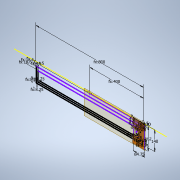
# Autodesk Inventor part: primary_coil_0R2_test_cut
Saved by Autodesk Inventor 2021 (Build 250183000, 183)
## iProperties
Created: 2021-01-20
Part Number: primary_coil_0R2_test_cut
Material: Generic
Document SubType Name: Modeling
Designer: phamv
Density: 1 g/cm^3
Appearance: Default
Author: phamv
Autodesk Inventor part; units mm, degrees
ref_plane "YZ Plane" through (0, 0, 0) normal (1, 0, 0) x (0, 1, 0)
sketch "Sketch1" plane through (0, 0, 0) normal (0, 0, 1) x (1, 0, 0)
  line L0 (-5, -4.3) -> (380, -4.3)
  line L1 (400, -24.3) -> (400, -120)
  line L2 (380, -140) -> (-400, -140)
  line L3 (-400, -140) -> (-400, -27.4)
  line L4 (-5, -4.3) -> (-5, -8.8)
  line L5 (-5, -8.8) -> (375.5, -8.8)
  line L6 (395.5, -28.8) -> (395.5, -115.5)
  line L7 (375.5, -135.5) -> (-395.5, -135.5)
  line L8 (-400, -27.4) -> (367.25, -27.4)
  line L9 (387.25, -47.4) -> (387.25, -107.25)
  line L10 (367.25, -127.25) -> (-387.25, -127.25)
  line L11 (-395.5, -135.5) -> (-395.5, -31.9)
  line L12 (-395.5, -31.9) -> (362.75, -31.9)
  line L13 (382.75, -51.9) -> (382.75, -102.75)
  line L14 (362.75, -122.75) -> (-382.75, -122.75)
  line L15 (-382.75, -122.75) -> (-382.75, -55)
  line L16 (-387.25, -127.25) -> (-387.25, -50.5)
  line L17 (-387.25, -50.5) -> (354.5, -50.5)
  line L18 (374.5, -70.5) -> (374.5, -94.5)
  line L19 (-382.75, -55) -> (350, -55)
  line L20 (370, -75) -> (370, -90)
  line L21 (350, -110) -> (-374.5, -110)
  line L22 (354.5, -114.5) -> (-374.5, -114.5)
  line L23 (-374.5, -114.5) -> (-374.5, -110)
  arc A0 (400, -24.3) -> (380, -4.3) centre (380, -24.3) ccw
  arc A1 (395.5, -28.8) -> (375.5, -8.8) centre (375.5, -28.8) ccw
  arc A2 (387.25, -47.4) -> (367.25, -27.4) centre (367.25, -47.4) ccw
  arc A3 (382.75, -51.9) -> (362.75, -31.9) centre (362.75, -51.9) ccw
  arc A4 (374.5, -70.5) -> (354.5, -50.5) centre (354.5, -70.5) ccw
  arc A5 (370, -75) -> (350, -55) centre (350, -75) ccw
  arc A6 (350, -110) -> (370, -90) centre (350, -90) ccw
  arc A7 (354.5, -114.5) -> (374.5, -94.5) centre (354.5, -94.5) ccw
  arc A8 (362.75, -122.75) -> (382.75, -102.75) centre (362.75, -102.75) ccw
  arc A9 (367.25, -127.25) -> (387.25, -107.25) centre (367.25, -107.25) ccw
  arc A10 (375.5, -135.5) -> (395.5, -115.5) centre (375.5, -115.5) ccw
  arc A11 (380, -140) -> (400, -120) centre (380, -120) ccw
  line L24 (323.0472, 0) -> (323.0472, -162)
  line L25 (323.0472, -162) -> (407.7972, -162)
  line L26 (407.7972, -162) -> (407.7972, 0)
  line L27 (407.7972, 0) -> (323.0472, 0)
  line L28 (-561.5594, 0) -> (569.3566, 0) projected
  line L29 (323.0472, -123.614) -> (323.0472, -67.5)
  line L30 (323.0472, -60) -> (345.0535, -60)
  line L31 (365.0535, -80) -> (365.0535, -85)
  line L32 (345.0535, -105) -> (323.0472, -105)
  arc A12 (365.0535, -62) -> (363.0535, -60) centre (363.0535, -62) ccw
  arc A13 (365.0535, -80) -> (345.0535, -60) centre (345.0535, -80) ccw
  arc A14 (345.0535, -105) -> (365.0535, -85) centre (345.0535, -85) ccw
  line L33 (323.0472, -13.3) -> (377.5888, -13.3)
  line L34 (377.5888, -13.3) -> (377.5888, -22.9)
  line L35 (377.5888, -22.9) -> (323.0472, -22.9)
  line L36 (323.0472, -36.4) -> (367.1423, -36.4)
  line L37 (367.1423, -36.4) -> (367.1423, -46)
  line L38 (367.1423, -46) -> (323.0472, -46)
  point P0 (0, 0)
  point P1 (400, -4.3)
  point P2 (400, -140)
  point P3 (395.5, -8.8)
  point P4 (395.5, -135.5)
  point P5 (387.25, -27.4)
  point P6 (387.25, -127.25)
  point P7 (382.75, -31.9)
  point P8 (382.75, -122.75)
  point P9 (374.5, -50.5)
  point P10 (374.5, -114.5)
  point P11 (370, -55)
  point P12 (370, -110)
  point P13 (0, 0)
  point P14 (323.0472, -55)
  point P15 (323.0472, -110)
  point P16 (323.0472, -31.9)
  point P17 (323.0472, -50.5)
  point P18 (323.0472, -114.5)
  point P19 (323.0472, -122.75)
  point P20 (323.0472, -8.8)
  point P21 (323.0472, -27.4)
  point P22 (323.0472, -127.25)
  point P23 (323.0472, -135.5)
  point P24 (323.0472, -140)
  point P25 (323.0472, -4.3)
  point P26 (323.0472, -52.3952)
  point P27 (323.0472, -58.8956)
  point P28 (323.0472, -28.1781)
  point P29 (323.0472, -37.5605)
  point P30 (365.0535, -60)
  point P31 (365.0535, -105)
  point P32 (323.0472, -105)
  dimension "d1" = 4.5
  dimension "d2" = 4.5
  dimension "d3" = 4.5
  dimension "d5" = 800
  dimension "d6" = 400
  dimension "d7" = 4.5
  dimension "d8" = 4.5
  dimension "d9" = 8.25
  dimension "d10" = 4.5
  dimension "d11" = 18.6
  dimension "d12" = 4.5
  dimension "d13" = 8.25
  dimension "d14" = 4.5
  dimension "d15" = 4.5
  dimension "d16" = 4.5
  dimension "d17" = 8.25
  dimension "d19" = 18.6
  dimension "d20" = 8.25
  dimension "d88" = 4.5
  dimension "d89" = 8.25
  dimension "d90" = 8.25
  dimension "d91" = 20
  dimension "d104" = 84.75
  dimension "d106" = 162
  dimension "d111" = 5
  dimension "d112" = 5
  dimension "d113" = 2
  dimension "d114" = 20
  dimension "d115" = 4.5
  dimension "d116" = 4.5
  dimension "d117" = 4.5
  dimension "d118" = 4.5
  dimension "d119" = 140
  constraints: 74 end point, 31 point on line, 30 point on circle, 30 tangent, 18 perpendicular, 15 centre point, 12 equal radius, 11 horizontal, 4 vertical, 2 parallel, 1 coincident, 1 collinear, 13 other
  measures "d1" distance between parallel lines of L5 L0
  measures "d2" distance between parallel lines of L6 L1
  measures "d3" distance between parallel lines of L2 L7
  measures "d5" distance between parallel lines of L3 L1
  measures "d6" distance from line of point (0, 0) L1
  measures "d7" distance between parallel lines of L3 L11
  measures "d8" distance between parallel lines of L13 L9
  measures "d9" distance between parallel lines of L9 L6
  measures "d10" distance between parallel lines of L8 L12
  measures "d11" distance between parallel lines of L8 L5
  measures "d12" distance between parallel lines of L10 L14
  measures "d13" distance between parallel lines of L7 L10
  measures "d14" distance between parallel lines of L16 L15
  measures "d15" distance between parallel lines of L17 L19
  measures "d16" distance between parallel lines of L20 L18
  measures "d17" distance between parallel lines of L18 L13
  measures "d19" distance between parallel lines of L17 L12
  measures "d20" distance between parallel lines of L11 L16
  measures "d88" distance between parallel lines of L22 L21
  measures "d89" distance between parallel lines of L14 L22
  measures "d90" distance between parallel lines of L15 L23
  measures "d91" radius of A0
  measures "d106" distance between parallel lines of L25 L27
  measures "d111" distance between parallel lines of L19 L30
  measures "d112" distance between parallel lines of L21 L32
  measures "d113" radius of A12
  measures "d114" radius of A13
  measures "d115" distance between parallel lines of L5 L33
  measures "d116" distance between parallel lines of L8 L35
  measures "d117" distance between parallel lines of L12 L36
  measures "d118" distance between parallel lines of L17 L38
  measures "d119" distance between parallel lines of L2 L28
extrude "Extrusion1" add sketch "Sketch1" along normal blind 4.5 contours L24 L27 L26 L25 L2 A11 L1 A0 L0 | L5 A1 L6 A10 L7 L24 L10 A9 L9 A2 L8 L35 L34 L33 | L12 A3 L13 A8 L14 L24 L22 A7 L18 A4 L17 L38 L37 L36 | L19 A5 L20 A6 L21 L24 L32 A14 L31 A13 L30
extrude "Extrusion7" add sketch "Sketch1" against normal blind 0.45 contours L24 L27 L26 L25 L2 A11 L1 A0 L0 | L0 A0 L1 A11 L2 L24 L7 A10 L6 A1 L5 | L5 A1 L6 A10 L7 L24 L10 A9 L9 A2 L8 L35 L34 L33 | L33 L34 L35 L24 | L8 A2 L9 A9 L10 L24 L14 A8 L13 A3 L12 | L12 A3 L13 A8 L14 L24 L22 A7 L18 A4 L17 L38 L37 L36 | L36 L37 L38 L24 | L17 A4 L18 A7 L22 L24 L21 A6 L20 A5 A12 L19 | L19 A5 L20 A6 L21 L24 L32 A14 L31 A13 L30 | L30 A13 L31 A14 L32 L24 | A12 A5
equation "\"d1\" = wire_diameter"
equation "\"d2\" = wire_diameter"
equation "\"d3\" = wire_diameter"
equation "\"d5\" = track_length"
equation "\"d6\" = 0.5 * track_length"
equation "\"d7\" = wire_diameter"
equation "\"d8\" = wire_diameter"
equation "\"d9\" = distance_between_wires_edge"
equation "\"d10\" = wire_diameter"
equation "\"d11\" = distance_between_wires"
equation "\"d12\" = wire_diameter"
equation "\"d13\" = distance_between_wires_edge"
equation "\"d14\" = wire_diameter"
equation "\"d15\" = wire_diameter"
equation "\"d16\" = wire_diameter"
equation "\"d17\" = distance_between_wires_edge"
equation "\"d19\" = distance_between_wires"
equation "\"d20\" = distance_between_wires_edge"
equation "\"d22\" = wire_diameter"
equation "\"track_length\" = 800"
equation "\"wire_diameter\" = 4.5"
equation "\"distance_between_wires\" = -1.2 * wire_diameter + 0.2 * parameter_6"
equation "\"distance_between_wires_edge\" = 8.25"
equation "\"parameter_6\" = 120"
body "Solid1"
